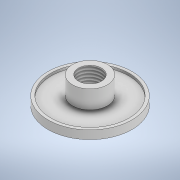
# Autodesk Inventor part: FLANCHE
Saved by Autodesk Inventor 2022 (Build 260153000, 153)
## iProperties
Created: 2022-09-01
Part Number: FLANCHE
Material: Genérico
Document SubType Name: Modeling
Designer: Usuario
Density: 1 g/cm^3
Appearance: Valor por defecto
Author: Usuario
Autodesk Inventor part; units mm, degrees
ref_plane "YZ Plane" through (0, 0, 0) normal (1, 0, 0) x (0, 1, 0)
ref_plane "XZ Plane" through (0, 0, 0) normal (0, 1, 0) x (-1, 0, 0)
ref_plane "XY Plane" through (0, 0, 0) normal (0, 0, 1) x (1, 0, 0)
sketch "Boceto1" plane through (0, 0, 0) normal (0, 1, 0) x (-1, 0, 0)
  circle A0 centre (0, 0) radius 34.6
  circle A1 centre (0, 0) radius 9.485
  circle A2 centre (0, 0) radius 14.45
  dimension "d0" = 69.2
  dimension "d1" = 18.97
  dimension "d2" = 28.9
  constraints: 3 centre point, 3 coincident
  measures "d0" diameter of A0
  measures "d1" diameter of A1
  measures "d2" diameter of A2
extrude "Extrusión1" add sketch "Boceto1" along normal blind 21.97 contours A2
extrude "Extrusión2" add sketch "Boceto1" along normal blind 6.95 contours A0
thread "Rosca1" size "M20x2.5" class "6H" standard "ANSI Metric M Profile" full length
sketch "Boceto2" plane through (0, 6.95, 0) normal (0, 1, 0) x (1, 0, 0)
  circle A0 centre (0, 0) radius 32.15
  dimension "d9" = 64.3
  constraints: 1 centre point, 1 coincident
  measures "d9" diameter of A0
extrude "Extrusión3" cut sketch "Boceto2" against normal blind 2
